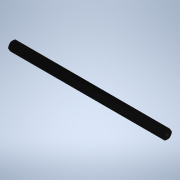
# Autodesk Inventor part: ABLSBF7-133-M3-N3
Saved by Autodesk Inventor 2020.4 (Build 244396000, 396)
## iProperties
Part Number: ABLSBF7-133-M3-N3
Material: 一般
Catalog Web Link: www.cadenas.de
Description: NLSBF, LSBF, PLSBF, BLSBF, SLSBF, ALSBF, ABLSBF-Hex Posts - Both Ends Tapped - L Dimension, Thread Dia. Configurable -
Vendor: MISUMI
Document SubType Name: Modeling
Designer: partserver
Manufacturer: MISUMI
Mass: 5.56155 g
Surface Area: 34.3327 cm^2
Volume: 5.56155 cm^3
Density: 1 g/cm^3
Appearance: 光沢 - 黒
Category: PARTsolutions
Company: MISUMI
PSOL_IDENT_0: {$CADENAS_DATA\23d-libs\misumi\metric\19_posts_stands\plsbf.prj},252 {VTYP=3D},{NB=ABLSBF7-133-M3-N3
PSOL_IDENT_1: },{LINA=ABLSBF7-133-M3-N3},{NN=NLSBF, LSBF, PLSBF, BLSBF, SLSBF, ALSBF, ABLSBF},{DATE=19.10.2021 02:
PSOL_IDENT_2: 45:16},{GEOMDATE=15.10.2021 09:43:14},{VERSION=},{LINEID=50},{WBVAR=MAT,ST,M,N,ALT1,L,ALT4,ALT2,ALT3
PSOL_IDENT_3: },{WBNUMERIC=M,N,L}  {NB=ABLSBF7-133-M3-N3},{LINA=ABLSBF7-133-M3-N3},{KT=DUMMY},{PN=ABLSBF7-133-M3-N
PSOL_IDENT_4: 3},{TYPE=ABLSBF},{MAT=A2011},{MATALG= 'LCS','Low Carbon Steel','304','SUS304','A2011','A2011-T8 Alum
PSOL_IDENT_5: inum Alloy' },{ST=BA},{STALG= 'CA','Clear Anodizing','BA','Black Anodizing'},{B=7},{M=3},{MALG=[3,4,
PSOL_IDENT_6: 5]},{N=3},{NALG=[3,4,5]},{ALT1=},{L=133.0},{LALG=[15:200/0.5]},{LMIN=15},{LMIN1=12},{LMIN1ALG=12},{L
PSOL_IDENT_7: MIN2=15.000},{C=8.1},{ALT4=},{ALT4ALG= '','Not applicable' },{ALT4PN=},{ALT2=},{ALT2ALG='','w/o MD (
PSOL_IDENT_8: Left End Change The Effective Tap Depth)','MD','with MD (Left End Change The Effective Tap Depth)'},
PSOL_IDENT_9: {ALT2PN=},{ALT3=},{ALT3ALG='','w/o ND (Right End Change The Effective Tap Depth)','ND','with ND (Rig
PSOL_IDENT_10: ht End Change The Effective Tap Depth)'},{ALT3PN=},{MAV=3},{MPITCH=0.5},{NPITCH=0.5},{NDEPT=9},{MDEP
PSOL_IDENT_11: T=9},{M3D=6},{N3D=6}
NB: ABLSBF7-133-M3-N3
NN: NLSBF, LSBF, PLSBF, BLSBF, SLSBF, ALSBF, ABLSBF
NT: Hex Posts - Both Ends Tapped - L Dimension, Thread Dia. Configurable -
NBSYN: $PN.
LINA: ABLSBF7-133-M3-N3
CATALOG: Misumi
PN: ABLSBF7-133-M3-N3
MAT: A2011-T8 Aluminum Alloy
ST: Black Anodizing
B: 7
M: 3
N: 3
ALT1: w/o LKC (L Dimension Tolerance)
L: 133
C: 8.1
ALT4: Not applicable
ALT2: w/o MD (Left End Change The Effective Tap Depth)
ALT3: w/o ND (Right End Change The Effective Tap Depth)
SUPPLIER: MISUMI
ARTICLENO: ABLSBF7-133-M3-N3
BOMINFO: ABLSBF7-133-M3-N3
CREATOR: CADENAS GmbH
Title: ABLSBF7-133-M3-N3
Author: Cadenas PARTsolutions
Comments: Hex Posts - Both Ends Tapped - L Dimension, Thread Dia. Configurable -
Autodesk Inventor part; units mm, degrees
sketch "Sketch_1" plane through (0, 0, 0) normal (0, 0, 1) x (1, 0, 0)
  line L0 (133, 0) -> (0, 0)
  line L1 (0, 0) -> (0, 3.5)
  line L2 (0, 3.5) -> (0.6062, 4.55)
  line L3 (0.6062, 4.55) -> (132.3938, 4.55)
  line L4 (132.3938, 4.55) -> (133, 3.5)
  line L5 (133, 3.5) -> (133, 0)
  line L6 (133, 0) -> (0, 0)
  constraints: 14 end point
revolve "Revolution1" add sketch "Sketch_1" angle 360 about axis through (133, 0, 0) along (1, 0, 0)
sketch "Sketch_2" plane through (0, 0, 0) normal (1, 0, 0) x (0, 1, 0)
  line L0 (7, 7) -> (-7, 7)
  line L1 (-7, 7) -> (-7, -7)
  line L2 (-7, -7) -> (7, -7)
  line L3 (7, -7) -> (7, 7)
  line L4 (-2.0207, 3.5) -> (-4.0415, 0)
  line L5 (-4.0415, 0) -> (-2.0207, -3.5)
  line L6 (-2.0207, -3.5) -> (2.0207, -3.5)
  line L7 (2.0207, -3.5) -> (4.0415, 0)
  line L8 (4.0415, 0) -> (2.0207, 3.5)
  line L9 (2.0207, 3.5) -> (-2.0207, 3.5)
  constraints: 20 end point
extrude "Extrusion1" cut sketch "Sketch_2" along normal blind 133
sketch "Sketch3" plane through (0, 0, 0) normal (-1, 0, 0) x (0, 0, 1)
  point P0 (0, 0)
hole "Hole1" at (0, 0, 0) direction (1, 0, 0) diameter 2.459 depth 8.2901 tip angle 120 countersink diameter 3 countersink angle 90 thread size "M3x0.5" class "6H" standard "ISO Metric profile"
sketch "Sketch4" plane through (133, 0, 0) normal (1, 0, 0) x (0, 0, -1)
  point P0 (0, 0)
hole "Hole2" at (133, 0, 0) direction (-1, 0, 0) diameter 2.459 depth 8.2901 tip angle 120 countersink diameter 3 countersink angle 90 thread size "M3x0.5" class "6H" standard "ISO Metric profile"
ref_plane "C3_XY" through (133, 0, 0) normal (-1, 0, 0) x (0, 0, -1)
ref_plane "C3_YZ" through (133, 0, 0) normal (0, 0, -1) x (0, -1, 0)
ref_plane "C3_ZX" through (133, 0, 0) normal (0, -1, 0) x (-1, 0, 0)
body "Solid1"
